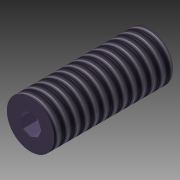
# Autodesk Inventor part: M2x6_D963
Saved by Autodesk Inventor 2015 (Build 190159000, 159)
## iProperties
Created: 2015-01-10
Part Number: M2x6_D963
Material: Generic
Document SubType Name: Modeling
Designer: ice
Density: 1 g/cm^3
Appearance: Default
Mass: 0.0153643 g
Surface Area: 0.393523 cm^2
Volume: 0.0153643 cm^3
Author: ice
Autodesk Inventor part; units mm, degrees
ref_plane "YZ Plane" through (0, 0, 0) normal (1, 0, 0) x (0, 1, 0)
ref_plane "Work Plane4" through (0, 0, 0) normal (0, -1, 0) x (1, 0, 0)
ref_plane "Work Plane10" through (0, 7.6, 0) normal (0, 1, 0) x (1, 0, 0)
sketch "Sketch7" plane through (0, 7.6, 0) normal (0, 1, 0) x (1, 0, 0)
  circle A0 centre (0, 0) radius 1
  constraints: 1 centre point, 1 coincident
extrude "Extrusion7" add sketch "Sketch7" against normal blind 5
sketch "Sketch8" plane through (0, 2.6, 0) normal (0, -1, 0) x (1, 0, 0)
  line L0 (0.45, 0) -> (0.3182, -0.3182)
  line L1 (0.3182, -0.3182) -> (0, -0.45)
  line L2 (0, -0.45) -> (-0.3182, -0.3182)
  line L3 (-0.3182, -0.3182) -> (-0.45, 0)
  line L4 (-0.45, 0) -> (-0.3182, 0.3182)
  line L5 (-0.3182, 0.3182) -> (0, 0.45)
  line L6 (0, 0.45) -> (0.3182, 0.3182)
  line L7 (0.3182, 0.3182) -> (0.45, 0)
  point P0 (0, 0)
  constraints: 16 end point, 2 perpendicular
extrude "Extrusion8" cut sketch "Sketch8" against normal blind 0.6
thread "Thread4" size "M2x0.4" class "6g" standard "ANSI Metric M Profile" full length
body "Solid2"
